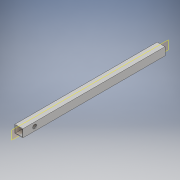
# Autodesk Inventor part: 2inSquareArmTube
Saved by Autodesk Inventor 2018.2 (Build 222227000, 227)
## iProperties
Created: 2018-02-07
Part Number: 2inSquareArmTube
Material: Generic
Document SubType Name: Modeling
Designer: steele
Density: 1 g/cm^3
Appearance: Default
Author: steele
Autodesk Inventor part; units mm, degrees
ref_plane "XZ Plane" through (0, 0, 0) normal (0, 1, 0) x (-1, 0, 0)
ref_plane "XY Plane" through (0, 0, 0) normal (0, 0, 1) x (1, 0, 0)
sketch "Sketch1" plane through (0, 0, 0) normal (0, 0, 1) x (1, 0, 0)
  line L0 (-25.4, -25.4) -> (25.4, -25.4)
  line L1 (25.4, -25.4) -> (25.4, 25.4)
  line L2 (25.4, 25.4) -> (-25.4, 25.4)
  line L3 (-25.4, 25.4) -> (-25.4, -25.4)
  line L4 (-25.4, -25.4) -> (25.4, 25.4) construction
  line L5 (25.4, -25.4) -> (-25.4, 25.4) construction
  line L6 (-22.225, -22.225) -> (22.225, -22.225)
  line L7 (22.225, -22.225) -> (22.225, 22.225)
  line L8 (22.225, 22.225) -> (-22.225, 22.225)
  line L9 (-22.225, 22.225) -> (-22.225, -22.225)
  line L10 (-22.225, -22.225) -> (22.225, 22.225) construction
  line L11 (22.225, -22.225) -> (-22.225, 22.225) construction
  point P0 (0, 0)
  dimension "d0" = 50.8
  dimension "d1" = 3.175
  constraints: 24 end point, 4 midpoint, 4 parallel, 4 perpendicular, 2 horizontal
  measures "d0" distance of L0.start L0.end
  measures "d1" distance between parallel lines of L6 L0
extrude "Extrusion1" add sketch "Sketch1" against normal blind 914.4
sketch "Sketch2" plane through (25.4, -25.4, 0) normal (1, 0, 0) x (0, 0, -1)
  circle A0 centre (76.2, 25.4) radius 12.7
  line L0 (0, 0) -> (0, 50.8) projected
  point P0 (0, 25.4)
  dimension "d4" = 25.4
  dimension "d7" = 76.2
  constraints: 1 centre point
  measures "d4" diameter of A0
  measures "d7" distance from line of A0.centre L0
extrude "Extrusion2" cut sketch "Sketch2" against normal through all
body "Solid1"
